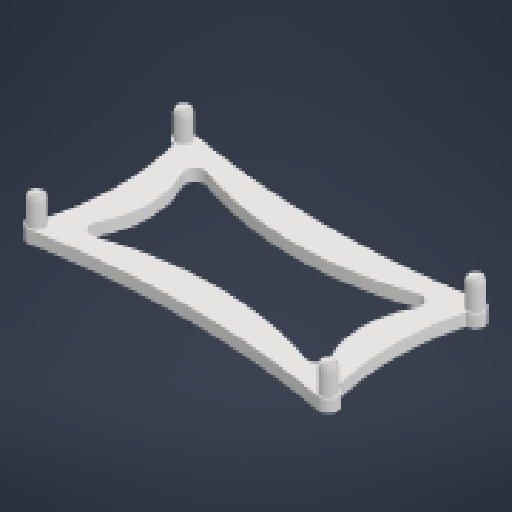
# Autodesk Inventor part: Esp32_Holder
Saved by Autodesk Inventor 2024 (Build 280153000, 153)
## iProperties
Created: 2023-10-16
Part Number: Esp32_Holder
Material: Generic
Document SubType Name: Modeling
Designer: 21guslof
Density: 1 g/cm^3
Appearance: Default
Author: 21guslof
Autodesk Inventor part; units mm, degrees
ref_plane "YZ Plane" through (0, 0, 0) normal (1, 0, 0) x (0, 1, 0)
ref_plane "XZ Plane" through (0, 0, 0) normal (0, 1, 0) x (-1, 0, 0)
ref_plane "XY Plane" through (0, 0, 0) normal (0, 0, 1) x (1, 0, 0)
sketch "Sketch1" plane through (0, 0, 0) normal (0, 1, 0) x (-1, 0, 0)
  circle A0 centre (0, 0) radius 1.5
  circle A1 centre (46.7, 0) radius 1.5
  circle A2 centre (46.7, 23.55) radius 1.5
  circle A3 centre (0, 23.55) radius 1.5
  circle A4 centre (46.7, 23.55) radius 1.25
  circle A5 centre (46.7, 0) radius 1.25
  circle A6 centre (0, 23.55) radius 1.25
  circle A7 centre (0, 0) radius 1.25
  arc A8 (0, 25.05) -> (46.7, 25.05) centre (23.35, 149.277457) ccw
  arc A9 (46.7, -1.5) -> (0, -1.5) centre (23.35, -125.727457) ccw
  arc A10 (46.7, 22.05) -> (46.7, 1.5) centre (85.443675, 11.775) ccw
  arc A11 (0, 1.5) -> (0, 22.05) centre (-38.743675, 11.775) ccw
  arc A12 (1.339339, 22.874595) -> (45.360661, 22.874595) centre (23.35, 68.821516) ccw
  arc A13 (45.360661, 22.874595) -> (45.360661, 0.675405) centre (55.180762, 11.775) ccw
  arc A14 (1.339339, 0.675405) -> (1.339339, 22.874595) centre (-8.480762, 11.775) ccw
  arc A15 (45.360661, 0.675405) -> (1.339339, 0.675405) centre (23.35, -45.271516) ccw
  arc A16 (6.339339, 20.798332) -> (5.025915, 17.874595) centre (5.377341, 19.473606) ccw
  arc A17 (41.674085, 17.874595) -> (40.360661, 20.798332) centre (41.322659, 19.473606) ccw
  arc A18 (40.360661, 2.751668) -> (41.674085, 5.675405) centre (41.322659, 4.076394) ccw
  arc A19 (5.025915, 5.675405) -> (6.339339, 2.751668) centre (5.377341, 4.076394) ccw
  point P0 (3.834051, 20.020045)
  point P1 (5.492596, 21.106718)
  point P2 (41.207404, 21.106718)
  point P3 (42.865949, 20.020045)
  point P4 (42.865949, 3.529955)
  point P5 (41.207404, 2.443282)
  point P6 (5.492596, 2.443282)
  point P7 (3.834051, 3.529955)
  point P8 (0.538581, 24.949975)
  point P9 (46.161419, -1.399975)
  dimension "d0" = 3
  dimension "d1" = 3
  dimension "d2" = 3
  dimension "d3" = 3
  dimension "d4" = 20.55
  dimension "d5" = 20.55
  dimension "d6" = 43.7
  dimension "d7" = 2.5
  dimension "d8" = 2.5
  dimension "d9" = 2.5
  dimension "d10" = 2.5
  constraints: 39 point on circle, 20 centre point, 5 coincident
  measures "d0" diameter of A0
  measures "d1" diameter of A1
  measures "d2" diameter of A2
  measures "d3" diameter of A3
  measures "d7" diameter of A4
  measures "d8" diameter of A5
  measures "d9" diameter of A6
  measures "d10" diameter of A7
extrude "Extrusion1" add sketch "Sketch1" along normal blind 2 contours A0 A9 | A0 A15 A19 A18 A1 A9 | A0 A11 A3 A14 A16 A19 | A14 A19 A15 | A19 A14 | A15 A19 | A9 A1 | A1 A9 | A3 A8 | A13 A18 A17 A2 A10 A1 | A15 A18 A13 | A3 A8 | A3 A8 A2 A12 A17 A16 | A12 A16 A14 | A16 A14 | A15 A18 | A13 A18 | A16 A12 | A2 A8 | A13 A17 A12 | A13 A17 | A17 A12 | A4 | A5 | A6 | A7 picked at (1.402251, -0.119195) picked at (45.729521, 24.569318)
fillet "Fillet1" radius 1.5 8 edges at (-42.8659, 1, 20.02) (-42.8659, 1, 3.53) (-41.2074, 1, 2.4433) (-41.2074, 1, 21.1067) (-3.8341, 1, 3.53) (-5.4926, 1, 2.4433) (-3.8341, 1, 20.02) (-5.4926, 1, 21.1067)
sketch "Sketch2" plane through (0, 2, 0) normal (0, 1, 0) x (1, 0, 0)
  arc A0 (0, -1.5) -> (0, 1.5) centre (0, 0) ccw
  circle A1 centre (0, 0) radius 1.25
  arc A2 (-0.538581, -24.949975) -> (0, -22.05) centre (0, -23.55) ccw
  circle A3 centre (0, -23.55) radius 1.25
  arc A4 (-46.7, -22.05) -> (-46.7, -25.05) centre (-46.7, -23.55) ccw
  circle A5 centre (-46.7, -23.55) radius 1.25
  arc A6 (-46.161419, 1.399975) -> (-46.7, -1.5) centre (-46.7, 0) ccw
  circle A7 centre (-46.7, 0) radius 1.25
  dimension "d23" = 2.5
  dimension "d24" = 2.5
  dimension "d25" = 2.5
  dimension "d26" = 2.5
  constraints: 4 centre point, 4 coincident
  measures "d23" diameter of A1
  measures "d24" diameter of A3
  measures "d25" diameter of A5
  measures "d26" diameter of A7
extrude "Extrusion2" add sketch "Sketch2" along normal blind 3.5
fillet "Fillet2" radius 1 4 edges at (-47.95, 5.5, 23.55) (-47.95, 5.5, 0) (-1.25, 5.5, 0) (-1.25, 5.5, 23.55)
move faces "Move1" translate (0, 1, 0) faces at (-46.271089, 4.649042, 24.712212) (-46.271089, 4.649042, 1.162212) (0.428911, 4.649042, 1.162212) (-0.428911, 4.649042, 24.712212)
body "Solid1"
